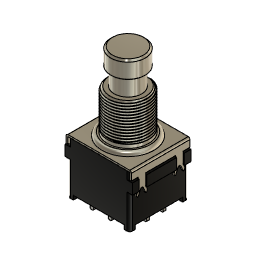
SF17010F-0302-21R-L (Autodesk Fusion 360 design; units mm, degrees)
Autodesk Fusion 360 part; units mm, degrees
ref_plane "WorkPlane1" through (0, 0, 1.2) normal (0, 0, 1) x (1, 0, 0)
sketch "Sketch1" plane through (0, 0, 1.2) normal (0, 0, 1) x (1, 0, 0)
  line L0 (-50, 50) -> (-30.4, 50)
  line L1 (-30.4, 50) -> (-30.4, 33)
  line L2 (-30.4, 33) -> (-50, 33)
  line L3 (-50, 33) -> (-50, 50)
  line L4 (-50, 50) -> (-30.4, 33) construction
  line L5 (-30.4, 50) -> (-50, 33) construction
  line L6 (9, -8.5) -> (-9, -8.5)
  line L7 (-9, -8.5) -> (-9, 8.5)
  line L8 (-9, 8.5) -> (9, 8.5)
  line L9 (9, 8.5) -> (9, -8.5)
  line L10 (9, -8.5) -> (-9, 8.5) construction
  line L11 (-9, -8.5) -> (9, 8.5) construction
  line L12 (-9, 8.5) -> (-7.4, 8.5)
  line L13 (-7.4, 8.5) -> (-7.4, 6.9)
  line L14 (-7.4, 6.9) -> (-9, 6.9)
  line L15 (-9, 6.9) -> (-9, 8.5)
  line L16 (-9, -8.5) -> (-7.4, -8.5)
  line L17 (-7.4, -8.5) -> (-7.4, -6.9)
  line L18 (-7.4, -6.9) -> (-9, -6.9)
  line L19 (-9, -6.9) -> (-9, -8.5)
  line L20 (9, -8.5) -> (7.4, -8.5)
  line L21 (7.4, -8.5) -> (7.4, -6.9)
  line L22 (7.4, -6.9) -> (9, -6.9)
  line L23 (9, -6.9) -> (9, -8.5)
  line L24 (9, 8.5) -> (7.4, 8.5)
  line L25 (7.4, 8.5) -> (7.4, 6.9)
  line L26 (7.4, 6.9) -> (9, 6.9)
  line L27 (9, 6.9) -> (9, 8.5)
  line L28 (1.7, -0.4) -> (-1.7, -0.4)
  line L29 (-1.7, -0.4) -> (-1.7, 0.4)
  line L30 (-1.7, 0.4) -> (1.7, 0.4)
  line L31 (1.7, 0.4) -> (1.7, -0.4)
  line L32 (1.7, -0.4) -> (-1.7, 0.4) construction
  line L33 (-1.7, -0.4) -> (1.7, 0.4) construction
  line L34 (-3.6, -4.4) -> (-3.6, -5.2)
  line L35 (-7, -4.4) -> (-3.6, -4.4)
  line L36 (-7, -5.2) -> (-7, -4.4)
  line L37 (-3.6, -5.2) -> (-7, -5.2)
  line L38 (1.7, -4.4) -> (1.7, -5.2)
  line L39 (-1.7, -4.4) -> (1.7, -4.4)
  line L40 (-1.7, -5.2) -> (-1.7, -4.4)
  line L41 (1.7, -5.2) -> (-1.7, -5.2)
  line L42 (7, -4.4) -> (7, -5.2)
  line L43 (3.6, -4.4) -> (7, -4.4)
  line L44 (3.6, -5.2) -> (3.6, -4.4)
  line L45 (7, -5.2) -> (3.6, -5.2)
  line L46 (-3.6, 0.4) -> (-3.6, -0.4)
  line L47 (-7, 0.4) -> (-3.6, 0.4)
  line L48 (-7, -0.4) -> (-7, 0.4)
  line L49 (-3.6, -0.4) -> (-7, -0.4)
  line L50 (7, 0.4) -> (7, -0.4)
  line L51 (3.6, 0.4) -> (7, 0.4)
  line L52 (3.6, -0.4) -> (3.6, 0.4)
  line L53 (7, -0.4) -> (3.6, -0.4)
  line L54 (-3.6, 5.2) -> (-3.6, 4.4)
  line L55 (-7, 5.2) -> (-3.6, 5.2)
  line L56 (-7, 4.4) -> (-7, 5.2)
  line L57 (-3.6, 4.4) -> (-7, 4.4)
  line L58 (1.7, 5.2) -> (1.7, 4.4)
  line L59 (-1.7, 5.2) -> (1.7, 5.2)
  line L60 (-1.7, 4.4) -> (-1.7, 5.2)
  line L61 (1.7, 4.4) -> (-1.7, 4.4)
  line L62 (7, 5.2) -> (7, 4.4)
  line L63 (3.6, 5.2) -> (7, 5.2)
  line L64 (3.6, 4.4) -> (3.6, 5.2)
  line L65 (7, 4.4) -> (3.6, 4.4)
  line L66 (0, 4.4) -> (0, 0.4) construction
  line L67 (0, -0.4) -> (0, -4.4) construction
  line L68 (7.5, 1.975) -> (-7.5, 1.975)
  line L69 (-7.5, 1.975) -> (-7.5, 2.825)
  line L70 (-7.5, 2.825) -> (7.5, 2.825)
  line L71 (7.5, 2.825) -> (7.5, 1.975)
  line L72 (7.5, 1.975) -> (-7.5, 2.825) construction
  line L73 (-7.5, 1.975) -> (7.5, 2.825) construction
  line L74 (7.5, -2.825) -> (-7.5, -2.825)
  line L75 (-7.5, -2.825) -> (-7.5, -1.975)
  line L76 (-7.5, -1.975) -> (7.5, -1.975)
  line L77 (7.5, -1.975) -> (7.5, -2.825)
  line L78 (7.5, -2.825) -> (-7.5, -1.975) construction
  line L79 (-7.5, -2.825) -> (7.5, -1.975) construction
  point P0 (-40.2, 41.5)
  point P1 (0, 2.4)
  point P2 (0, -2.4)
  point P3 (0, 2.4)
  point P4 (0, -2.4)
  dimension "d1" = 19.6
  dimension "d2" = 17
  dimension "d3" = 18
  dimension "d4" = 17
  dimension "d5" = 1.6
  dimension "d6" = 1.6
  dimension "d7" = 1.6
  dimension "d8" = 1.6
  dimension "d9" = 1.6
  dimension "d10" = 1.6
  dimension "d11" = 1.6
  dimension "d12" = 1.6
  dimension "d13" = 3.4
  dimension "d14" = 0.8
  dimension "d17" = 5.3
  dimension "d18" = 4.8
  dimension "d19" = 15
  dimension "d20" = 0.85
  dimension "d21" = 15
  dimension "d22" = 0.85
  constraint horizontal L0
  constraint vertical L1
  constraint horizontal L2
  constraint vertical L3
  constraint midpoint L4 P0
  constraint horizontal L6
  constraint perpendicular L6 L7
  constraint parallel L6 L8
  constraint parallel L7 L9
  constraint coincident L10 origin
  constraint coincident L11 origin
  constraint horizontal L12
  constraint vertical L13
  constraint horizontal L14
  constraint vertical L15
  constraint horizontal L16
  constraint vertical L17
  constraint horizontal L18
  constraint vertical L19
  constraint horizontal L20
  constraint vertical L21
  constraint horizontal L22
  constraint vertical L23
  constraint horizontal L24
  constraint vertical L25
  constraint horizontal L26
  constraint vertical L27
  constraint horizontal L28
  constraint perpendicular L28 L29
  constraint parallel L28 L30
  constraint parallel L29 L31
  constraint coincident L32 origin
  constraint coincident L33 origin
  constraint midpoint L61 L66.start
  constraint midpoint L30 L66.end
  constraint midpoint L66 P3
  constraint midpoint L28 L67.start
  constraint midpoint L39 L67.end
  constraint midpoint L67 P4
  constraint horizontal L68
  constraint perpendicular L68 L69
  constraint parallel L68 L70
  constraint parallel L69 L71
  constraint coincident L72 P3
  constraint coincident L73 P3
  constraint coincident P3 P1
  constraint horizontal L74
  constraint perpendicular L74 L75
  constraint parallel L74 L76
  constraint parallel L75 L77
  constraint coincident L78 P4
  constraint coincident L79 P4
  constraint coincident P4 P2
  measures "d1" distance of L0.start L0.end
  measures "d2" distance of L0.start L2.end
  measures "d3" distance of L7.end L8.end
  measures "d4" distance of L6.end L7.end
  measures "d5" distance of L7.end L12.end
  measures "d6" distance of L7.end L14.end
  measures "d7" distance of L6.end L16.end
  measures "d8" distance of L6.end L18.end
  measures "d9" distance of L6.start L20.end
  measures "d10" distance of L6.start L22.end
  measures "d11" distance of L8.end L24.end
  measures "d12" distance of L8.end L26.end
  measures "d13" distance of L29.end L30.end
  measures "d14" distance of L28.end L29.end
  measures "d19" distance of L69.end L70.end
  measures "d20" distance of L68.end L69.end
  measures "d21" distance of L75.end L76.end
  measures "d22" distance of L74.end L75.end
extrude "Extrude1" add sketch "Sketch1" against normal blind 1.2 contours L6 L9 L20 L21 L22 L23 | L6 L7 L16 L17 L18 L19 | L8 L9 L24 L25 L26 L27 | L7 L8 L12 L13 L14 L15 makes body 1 at (7.9333, 7.4333, 1.2) makes body 2 at (7.9333, -7.9667, 1.2) makes body 3 at (-7.9333, 7.4333, 1.2) makes body 4 at (-8.4667, -7.9667, 1.2)
extrude "Extrude2" add sketch "Sketch1" against normal blind 1 separate body contours L68 L69 L70 L71 | L74 L75 L76 L77 makes body 5 at (2.5, -2.825, 0.8667) makes body 6 at (2.5, 1.975, 0.8667)
extrude "Extrude3" add sketch "Sketch1" along normal blind 14 contours L6 L9 L20 L21 L22 L23 | L6 L7 L8 L9 L13 L14 L17 L18 L21 L22 L25 L26 | L6 L7 L16 L17 L18 L19 | L8 L9 L24 L25 L26 L27 | L7 L8 L12 L13 L14 L15 | L28 L29 L30 L31 | L34 L35 L36 L37 | L38 L39 L40 L41 | L42 L43 L44 L45 | L46 L47 L48 L49 | L50 L51 L52 L53 | L54 L55 L56 L57 | L58 L59 L60 L61 | L62 L63 L64 L65 | L68 L69 L70 L71 | L74 L75 L76 L77 bodies 1 2 3 4 5 6
ref_plane "WorkPlane2" through (-8.2, -7.7, 9.8) normal (0, 0, -1) x (-1, 0, 0)
sketch "Sketch2" plane through (-8.7, -7.7, 9.8) normal (0, 0, -1) x (1, 0, 0)
  line L0 (17.7, 0.8) -> (17.7, -16.2)
  line L1 (17.7, -16.2) -> (-0.3, -16.2)
  line L2 (-0.3, -16.2) -> (-0.3, 0.8)
  line L3 (-0.3, 0.8) -> (17.7, 0.8)
  line L4 (8.7, -16.2) -> (8.7, 0.8) construction
  line L5 (-1.1, -16.2) -> (-0.3, -16.2)
  line L6 (-1.1, -14.25) -> (-0.3, -14.25)
  line L7 (-0.3, -7.7) -> (17.7, -7.7) construction
  line L8 (-1.1, -12.05) -> (-0.3, -12.05)
  line L9 (-1.1, -16.2) -> (-1.1, -14.25)
  line L10 (-1.1, 0.8) -> (-0.3, 0.8)
  line L11 (-1.1, 0.8) -> (-1.1, -1.15)
  line L12 (-1.1, -1.15) -> (-0.3, -1.15)
  line L13 (-1.1, -3.35) -> (-0.3, -3.35)
  line L14 (-1.1, -12.05) -> (-1.1, -3.35)
  line L15 (-1.1, -1.15) -> (-1.1, 0.8)
  line L16 (18.5, -1.15) -> (17.7, -1.15)
  line L17 (18.5, -12.05) -> (18.5, -3.35)
  line L18 (17.7, -16.2) -> (17.7, 0.8)
  line L19 (18.5, 0.8) -> (18.5, -1.15)
  line L20 (18.5, -3.35) -> (17.7, -3.35)
  line L21 (18.5, -1.15) -> (18.5, 0.8)
  line L22 (18.5, -12.05) -> (17.7, -12.05)
  line L23 (18.5, -16.2) -> (18.5, -14.25)
  line L24 (18.5, 0.8) -> (17.7, 0.8)
  line L25 (18.5, -16.2) -> (17.7, -16.2)
  line L26 (18.5, -14.25) -> (17.7, -14.25)
  point P0 (-0.3, 0.8)
  point P1 (17.7, -7.7)
  point P2 (17.7, 0.8)
  dimension "d31" = 9.8
  dimension "d32" = 1.95
  dimension "d33" = 2.2
  constraint vertical L9
  constraint midpoint L1 L4.start
  constraint midpoint L3 L4.end
  constraint coincident L1 L5.start
  constraint coincident L3 L10.start
  constraint coincident L1.end L2.start
  constraint coincident L2 L6.end
  constraint perpendicular L2 L6
  constraint midpoint L2 L7.start
  constraint midpoint L0 P1
  constraint coincident L8.start L9
  constraint coincident L2 L8.end
  constraint perpendicular L2 L8
  constraint collinear L9 L14
  constraint symmetric L1.end L7 P0
  constraint symmetric L5.start L7 L10.start
  constraint symmetric L6.start L7 L11.end
  constraint symmetric L6.end L7 L12.end
  constraint symmetric L7 L8.start L13.start
  constraint symmetric L7 L8.end L13.end
  constraint collinear L14 L15
  constraint symmetric L1.end L4 L0.end
  constraint symmetric P0 L4 P2
  constraint symmetric L5.start L4 L23.start
  constraint symmetric L10.start L4 L19.start
  constraint symmetric L4 L1.end L0.end
  constraint symmetric L4 L6.start L23.end
  constraint symmetric L4 L6.end L26.end
  constraint symmetric L4 L7.start P1
  constraint symmetric L4 L8.start L17.start
  constraint symmetric L4 L8.end L22.end
  constraint symmetric L4 P0 P2
  constraint symmetric L4 L11.end L16.start
  constraint symmetric L4 L12.end L16.end
  constraint symmetric L4 L10.start L19.start
  constraint symmetric L4 L13.start L17.end
  constraint symmetric L4 L13.end L20.end
  measures "d31" distance of L4 L9
  measures "d32" distance of L5 L6
  measures "d33" distance of L6 L8
extrude "Extrude4" add sketch "Sketch2" against normal blind 3.1 contours L0 L16 L18 L19 L21 L24 | L2 L10 L11 L12 L15 | L0 L17 L18 L20 L22 | L2 L8 L13 L14 | L0 L18 L23 L25 L26 | L2 L5 L6 L9 bodies 1
sketch "Sketch3" plane through (0, 0, 15.2) normal (0, 0, 1) x (-1, 0, 0)
  line L0 (-9, -8.5) -> (9, -8.5)
  line L1 (9, 8.5) -> (-9, 8.5)
  line L2 (9.5, -8.5) -> (9.5, 8.5)
  line L3 (-9.5, 8.5) -> (-9.5, -8.5)
  line L4 (9.5, -8.5) -> (9, -8.5)
  line L5 (9.5, 8.5) -> (9, 8.5)
  line L6 (-9.5, 8.5) -> (-9, 8.5)
  line L7 (-9.5, -8.5) -> (-9, -8.5)
  line L8 (9, -8.5) -> (9, 8.5)
  line L9 (-9, 8.5) -> (-9, -8.5)
  constraint coincident L0.end L4.end
  constraint coincident L1.start L5.end
  constraint coincident L1.end L6.end
  constraint coincident L0.start L7.end
extrude "Extrude5" add sketch "Sketch3" along normal blind 0.5 separate body makes body 7
extrude "Extrude6" add sketch "Sketch3" against normal up to surface (1.95 mm away) contours L3 L6 L7 L9 | L2 L4 L5 L8 bodies 7
fillet "Fillet1" radius 0.5 2 edges at (-9.5, 0, 15.7) (9.5, 0, 15.7) on bodies 7
sketch "Sketch4" plane through (0, 0, 15.7) normal (0, 0, 1) x (-1, 0, 0)
  circle A0 centre (0, 0) radius 7.5
  line L0 (9, 8.5) -> (-9, 8.5)
  dimension "d44" = 1
  constraint coincident A0.centre origin
  measures "d44" distance of A0 L0
extrude "Extrude7" add sketch "Sketch4" along normal blind 1 bodies 7
fillet "Fillet2" radius 1 1 edges at (6.9925, 2.7121, 16.7) on bodies 7
sketch "Sketch5" plane through (0, 0, 16.7) normal (0, 0, 1) x (-1, 0, 0)
  circle A0 centre (0, 0) radius 6
  line L0 (-1, 0) -> (-1, -5.9161)
  line L1 (1, 0) -> (1, -5.9161)
  line L2 (1, -5) -> (-1, -5)
  line L3 (0, -5) -> (-0.75, -5)
  line L4 (-0.75, -5) -> (-0.75, -5.5)
  line L5 (-0.75, -5.5) -> (0.75, -5.5)
  line L6 (0.75, -5.5) -> (0.75, -5)
  line L7 (0.75, -5) -> (-0.1, -5)
  dimension "d49" = 12
  dimension "d50" = 2
  dimension "d51" = 1
  dimension "d52" = 0.75
  dimension "d53" = 0.5
  dimension "d54" = 1.5
  constraint coincident A0.centre origin
  constraint coincident A0 L0.end
  constraint vertical L0
  constraint coincident A0 L1.end
  constraint parallel L0 L1
  constraint coincident L1 L2.start
  constraint coincident L0 L2.end
  constraint perpendicular L0 L2
  constraint midpoint L2 L3.start
  constraint parallel L2 L3
  constraint perpendicular L2 L4
  constraint perpendicular L4 L5
  constraint coincident L2 L6.end
  constraint perpendicular L2 L6
  constraint coincident L3 L7.end
  constraint perpendicular L6 L7
  measures "d49" diameter of A0
  measures "d50" distance of L0 L1
  measures "d51" distance of A0 L2
  measures "d52" distance of L3.start L3.end
  measures "d53" distance of L3.end L4.end
  measures "d54" distance of L4.end L5.end
extrude "Extrude8" add sketch "Sketch5" along normal blind 0.8 contours L2 L3 L4 L5 L6 L7 bodies 7
fillet "Fillet3" radius 0.25 2 edges at (0.75, 5.25, 17.5) (-0.75, 5.25, 17.5) on bodies 7
extrude "Extrude9" add sketch "Sketch5" along normal blind 1 separate body contours A0 L0 L1 L2 L3 L7 makes body 8
sketch "Sketch8" plane through (0, 0, 17.7) normal (0, 0, 1) x (-1, 0, 0)
  circle A0 centre (0, 0) radius 6
  dimension "d72" = 12
  constraint coincident A0.centre origin
  measures "d72" diameter of A0
extrude "Extrude10" add sketch "Sketch8" 1 faces at (-0.1252, -2.3206, 17.7) along normal blind 10.5 separate body on bodies 8 makes body 9
thread "Thread1" "ISO Metric profile 12.0 M12x0.75 6g" major diameter 11.908 minor diameter 11.0445 pitch 0.75 angle 60 modelled right hand crest width 0.1036 on face at (-5.9925, 0.2991, 21.2) crest through (-5.954, 0, 17.5125) on bodies 9
sketch "Sketch7" plane through (0, 0, 28.2) normal (0, 0, 1) x (-1, 0, 0)
  circle A0 centre (0, 0) radius 6
  circle A1 centre (0, 0) radius 8
  dimension "d65" = 12
  dimension "d66" = 16
  constraint coincident A0.centre A1.centre
  measures "d65" diameter of A0
  measures "d66" diameter of A1
extrude "Extrude11" add sketch "Sketch7" against normal blind 0.8 separate body makes body 10
extrude "Extrude12" add sketch "Sketch7" along normal blind 1 contours A0 | A1 bodies 10
chamfer "Chamfer3" distance 0.8 angle 45 1 edges at (5.594, -2.1697, 28.2) on bodies 10
combine "Combine1" operation cut target body 9 tool bodies 10
move_body "Move1" bodies 9 to x (-0.5, 0.866025, 0) y (-0.866025, -0.5, 0) z (0, 0, 1) at (0, 0, 0)
extrude "Extrude13" cut sketch "Sketch5" along normal up to surface (11.5 mm away) contours A0 L0 L1 L2 L4 L5 L6 | L2 L3 L4 L5 L6 L7 bodies 9
combine "Combine2" operation add target body 9 tool bodies 8
sketch "Sketch9" plane through (0, 0, 28.2) normal (0, 0, 1) x (-1, 0, 0)
  circle A0 centre (0, 0) radius 4
  dimension "d75" = 8
  constraint coincident A0.centre origin
  measures "d75" diameter of A0
extrude "Extrude15" add 1 faces at (0, 1.3333, 16.7) along direction (0, 0, -1) up to surface (1.5 mm away) on bodies 9 bodies 9
extrude "Extrude16" cut sketch "Sketch9" against normal up to surface (13 mm away) bodies 7 9
combine "Combine3" operation cut target body 7 tool bodies 9 keep tools
sketch "Sketch10" plane through (0, 0, 15.2) normal (0, 0, -1) x (1, 0, 0)
  circle A0 centre (0, 0) radius 6
  dimension "d82" = 12
  constraint coincident A0.centre origin
  measures "d82" diameter of A0
extrude "Extrude17" cut sketch "Sketch10" against normal up to surface (1 mm away) bodies 7
extrude "Extrude18" add sketch "Sketch9" along normal blind 5 and the other way up to surface (13 mm away) separate body makes body 11
sketch "Sketch11" plane through (0, 0, 33.2) normal (0, 0, 1) x (-1, 0, 0)
  circle A0 centre (0, 0) radius 5
  dimension "d89" = 10
  constraint coincident A0.centre origin
  measures "d89" diameter of A0
extrude "Extrude19" add sketch "Sketch11" along normal blind 5 bodies 11
chamfer "Chamfer4" distance 0.5 angle 45 1 edges at (4.6616, 1.8081, 38.2) on bodies 11
chamfer "Chamfer4" distance 0.2 angle 45 1 edges at (4.6616, 1.8081, 33.2) on bodies 11
extrude "Extrude20" cut sketch "Sketch1" along normal blind 4 contours L28 L29 L30 L31 | L34 L35 L36 L37 | L38 L39 L40 L41 | L42 L43 L44 L45 | L46 L47 L48 L49 | L50 L51 L52 L53 | L54 L55 L56 L57 | L58 L59 L60 L61 | L62 L63 L64 L65 bodies 1
extrude "Extrude21" add sketch "Sketch1" along normal blind 4 separate body contours L28 L29 L30 L31 | L34 L35 L36 L37 | L38 L39 L40 L41 | L42 L43 L44 L45 | L46 L47 L48 L49 | L50 L51 L52 L53 | L54 L55 L56 L57 | L58 L59 L60 L61 | L62 L63 L64 L65 makes body 12 at (0.5667, -0.4, 2.5333) makes body 13 at (-4.7333, 4.4, 2.5333) makes body 14 at (0.5667, 4.4, 2.5333) makes body 15 at (0.5667, -5.2, 2.5333) makes body 16 at (4.7333, -0.4, 3.8667) makes body 17 at (-4.7333, -0.4, 2.5333) makes body 18 at (4.7333, 4.4, 3.8667) makes body 19 at (-4.7333, -5.2, 2.5333) makes body 20 at (4.7333, -5.2, 3.8667)
extrude "Extrude22" add 9 faces at (0.5667, 4.6667, 1.2) (5.8667, 4.6667, 1.2) (5.8667, -0.1333, 1.2) (0.5667, -0.1333, 1.2) (-4.7333, 4.6667, 1.2) (-4.7333, -0.1333, 1.2) (-4.7333, -4.9333, 1.2) (0.5667, -4.9333, 1.2) (5.8667, -4.9333, 1.2) along direction (0, 0, -1) blind 0.5 on bodies 12 13 14 15 16 17 18 19 20 bodies 14 12 13 15 16 17 18 19 20
sketch "Sketch12" plane through (0, 0, 0.7) normal (0, 0, -1) x (1, 0, 0)
  line L0 (0.5, -0.4) -> (-0.5, -0.4)
  line L1 (-0.5, -0.4) -> (-0.5, 0.4)
  line L2 (-0.5, 0.4) -> (0.5, 0.4)
  line L3 (0.5, 0.4) -> (0.5, -0.4)
  line L4 (0.5, -0.4) -> (-0.5, 0.4) construction
  line L5 (-0.5, -0.4) -> (0.5, 0.4) construction
  line L6 (-5.8, -5.2) -> (-4.8, -4.4) construction
  line L7 (-4.8, -5.2) -> (-5.8, -5.2)
  line L8 (-4.8, -4.4) -> (-4.8, -5.2)
  line L9 (-5.8, -4.4) -> (-4.8, -4.4)
  line L10 (-4.8, -5.2) -> (-5.8, -4.4) construction
  line L11 (-5.8, -5.2) -> (-5.8, -4.4)
  line L12 (-0.5, -5.2) -> (0.5, -4.4) construction
  line L13 (0.5, -5.2) -> (-0.5, -5.2)
  line L14 (0.5, -4.4) -> (0.5, -5.2)
  line L15 (-0.5, -4.4) -> (0.5, -4.4)
  line L16 (0.5, -5.2) -> (-0.5, -4.4) construction
  line L17 (-0.5, -5.2) -> (-0.5, -4.4)
  line L18 (4.8, -5.2) -> (5.8, -4.4) construction
  line L19 (5.8, -5.2) -> (4.8, -5.2)
  line L20 (5.8, -4.4) -> (5.8, -5.2)
  line L21 (4.8, -4.4) -> (5.8, -4.4)
  line L22 (5.8, -5.2) -> (4.8, -4.4) construction
  line L23 (4.8, -5.2) -> (4.8, -4.4)
  line L24 (-5.8, -0.4) -> (-4.8, 0.4) construction
  line L25 (-4.8, -0.4) -> (-5.8, -0.4)
  line L26 (-4.8, 0.4) -> (-4.8, -0.4)
  line L27 (-5.8, 0.4) -> (-4.8, 0.4)
  line L28 (-4.8, -0.4) -> (-5.8, 0.4) construction
  line L29 (-5.8, -0.4) -> (-5.8, 0.4)
  line L30 (4.8, -0.4) -> (5.8, 0.4) construction
  line L31 (5.8, -0.4) -> (4.8, -0.4)
  line L32 (5.8, 0.4) -> (5.8, -0.4)
  line L33 (4.8, 0.4) -> (5.8, 0.4)
  line L34 (5.8, -0.4) -> (4.8, 0.4) construction
  line L35 (4.8, -0.4) -> (4.8, 0.4)
  line L36 (-5.8, 4.4) -> (-4.8, 5.2) construction
  line L37 (-4.8, 4.4) -> (-5.8, 4.4)
  line L38 (-4.8, 5.2) -> (-4.8, 4.4)
  line L39 (-5.8, 5.2) -> (-4.8, 5.2)
  line L40 (-4.8, 4.4) -> (-5.8, 5.2) construction
  line L41 (-5.8, 4.4) -> (-5.8, 5.2)
  line L42 (-0.5, 4.4) -> (0.5, 5.2) construction
  line L43 (0.5, 4.4) -> (-0.5, 4.4)
  line L44 (0.5, 5.2) -> (0.5, 4.4)
  line L45 (-0.5, 5.2) -> (0.5, 5.2)
  line L46 (0.5, 4.4) -> (-0.5, 5.2) construction
  line L47 (-0.5, 4.4) -> (-0.5, 5.2)
  line L48 (4.8, 4.4) -> (5.8, 5.2) construction
  line L49 (5.8, 4.4) -> (4.8, 4.4)
  line L50 (5.8, 5.2) -> (5.8, 4.4)
  line L51 (4.8, 5.2) -> (5.8, 5.2)
  line L52 (5.8, 4.4) -> (4.8, 5.2) construction
  line L53 (4.8, 4.4) -> (4.8, 5.2)
  point P0 (-5.3, -4.8)
  point P1 (-5.3, -4.8)
  point P2 (0, -4.8)
  point P3 (0, -4.8)
  point P4 (5.3, -4.8)
  point P5 (5.3, -4.8)
  point P6 (-5.3, 0)
  point P7 (-5.3, 0)
  point P8 (5.3, 0)
  point P9 (5.3, 0)
  point P10 (-5.3, 4.8)
  point P11 (-5.3, 4.8)
  point P12 (0, 4.8)
  point P13 (0, 4.8)
  point P14 (5.3, 4.8)
  point P15 (5.3, 4.8)
  dimension "d100" = 1
  dimension "d101" = 0.8
  dimension "d104" = 5.3
  dimension "d105" = 4.8
  constraint horizontal L0
  constraint perpendicular L0 L1
  constraint parallel L0 L2
  constraint parallel L1 L3
  constraint coincident L4 origin
  constraint coincident L5 origin
  measures "d100" distance of L1.end L2.end
  measures "d101" distance of L0.end L1.end
extrude "Extrude23" add sketch "Sketch12" along normal up to surface (3.7 mm away) bodies 12 13 14 15 16 17 18 19 20
chamfer "Chamfer5" distance 0.4 angle 45 15 edges at (-5.8, 4.8, 0.7) (-4.8, 4.8, 0.7) (0.5, 0, 0.7) (-0.5, 0, 0.7) (-0.5, 4.8, 0.7) (0.5, 4.8, 0.7) (5.8, 0, 0.7) (0.5, -4.8, 0.7) (-0.5, -4.8, 0.7) (-5.8, 0, 0.7) (-4.8, 0, 0.7) (-5.8, -4.8, 0.7) (4.8, 4.8, 0.7) (5.8, 4.8, 0.7) (5.8, -4.8, 0.7) on bodies 12 13 14 15 16 17 18 19 20
fillet "Fillet6" radius 0.2 18 edges at (0.5, 0, -3) (-0.5, 0, -3) (-5.8, 4.8, -3) (-4.8, 4.8, -3) (0.5, 4.8, -3) (-0.5, 4.8, -3) (-0.5, -4.8, -3) (0.5, -4.8, -3) (4.8, 0, -3) (5.8, 0, -3) (-5.8, 0, -3) (-4.8, 0, -3) (4.8, 4.8, -3) (5.8, 4.8, -3) (-5.8, -4.8, -3) (-4.8, -4.8, -3) (4.8, -4.8, -3) (5.8, -4.8, -3) on bodies 12 13 14 15 16 17 18 19 20
sketch "Sketch14" plane through (-9, 0, 0) normal (-1, 0, 0) x (0, -1, 0)
  line L0 (-6.55, 9.8) -> (-6.55, 12.9)
  line L1 (-4.35, 9.8) -> (-4.35, 12.9)
  line L2 (8.5, 13.25) -> (-8.5, 13.25)
  line L3 (-6.55, 12.9) -> (-6.55, 13.25)
  line L4 (-4.35, 12.9) -> (-4.35, 13.25)
  line L5 (-6.55, 9.8) -> (-4.35, 9.8) construction
  line L6 (-5.4502, 10.2) -> (-5.4502, 7.9) construction
  line L7 (-6.6002, 8.194) -> (-5.8156, 9.9622)
  line L8 (-5.4502, 10.2) -> (-6.3831, 8.0977) construction
  line L9 (-6.3831, 8.0977) -> (-6.448, 8.1265) construction
  line L10 (-6.9561, 9.1178) -> (-6.55, 10.0331)
  line L11 (-6.6002, 8.194) -> (-6.6002, 8.194)
  arc A0 (-6.9561, 9.1178) -> (-6.6002, 8.194) centre (-6.3163, 8.8339) ccw
  line L12 (-3.9443, 9.1178) -> (-4.3504, 10.0331)
  arc A1 (-4.3002, 8.194) -> (-3.9443, 9.1178) centre (-4.5841, 8.8339) ccw
  line L13 (-4.3002, 8.194) -> (-5.0848, 9.9622)
  arc A2 (-5.0775, 9.9456) -> (-5.8156, 9.9622) centre (-5.45, 9.8) ccw
  line L14 (0, 13.25) -> (0, 7) construction
  line L15 (4.3002, 8.194) -> (5.0848, 9.9622)
  line L16 (6.6002, 8.194) -> (6.6002, 8.194)
  line L17 (3.9443, 9.1178) -> (4.3504, 10.0331)
  line L18 (4.35, 9.8) -> (4.35, 12.9)
  line L19 (6.55, 9.8) -> (6.55, 12.9)
  arc A3 (6.6002, 8.194) -> (6.9561, 9.1178) centre (6.3163, 8.8339) ccw
  line L20 (6.6002, 8.194) -> (5.8156, 9.9622)
  line L21 (5.4502, 10.2) -> (5.4502, 7.9) construction
  line L22 (6.55, 9.8) -> (4.35, 9.8) construction
  line L23 (5.4502, 10.2) -> (6.3831, 8.0977) construction
  line L24 (4.35, 12.9) -> (4.35, 13.25)
  line L25 (6.55, 12.9) -> (6.55, 13.25)
  line L26 (6.9561, 9.1178) -> (6.55, 10.0331)
  arc A4 (3.9443, 9.1178) -> (4.3002, 8.194) centre (4.5841, 8.8339) ccw
  line L27 (6.3831, 8.0977) -> (6.448, 8.1265) construction
  arc A5 (5.8156, 9.9622) -> (5.0775, 9.9456) centre (5.45, 9.8) ccw
  dimension "d123" = 0.8
  dimension "d127" = 2.3
  dimension "d128" = 1.15
  dimension "d130" = 0.7
  constraint coincident L0.end L3.start
  constraint coincident L2 L3.end
  constraint perpendicular L2 L3
  constraint coincident L1.end L4.start
  constraint coincident L2 L4.end
  constraint coincident L0.start L5.start
  constraint coincident L1.start L5.end
  constraint midpoint L5 A2.centre
  constraint perpendicular L5 L6
  constraint tangent L7 A2
  constraint coincident L6.start A2
  constraint parallel L7 L8
  constraint perpendicular L8 L9
  constraint collinear L7.start L8.end L9.end
  constraint parallel L7 L10
  constraint coincident L0 L10.end
  constraint tangent L10 A0
  constraint symmetric L6 L7.start A1.start
  constraint symmetric L6 L7.end L13.end
  constraint symmetric L6 L10.end L12.end
  constraint symmetric L6 L10.start L12.start
  constraint symmetric L6 A0 A1
  constraint coincident L13 A2.start
  constraint midpoint L2 L14.start
  constraint perpendicular L2 L14
  constraint symmetric L0.start L14 L19.start
  constraint symmetric L0.end L14 L19.end
  constraint symmetric L1.start L14 L18.start
  constraint symmetric L1.end L14 L18.end
  constraint symmetric L3.end L14 L25.end
  constraint symmetric L4.end L14 L24.end
  constraint symmetric L6.end L14 L21.end
  constraint symmetric L7.start L14 L16.start
  constraint symmetric L6.start L14 L21.start
  constraint symmetric L7.end L14 L20.end
  constraint symmetric L8.end L14 L23.end
  constraint symmetric L9.end L14 L27.end
  constraint symmetric L10.end L14 L26.end
  constraint symmetric L10.start L14 A3.end
  constraint symmetric A0 L14 A3
  constraint symmetric L12.start L14 L17.start
  constraint symmetric L12.end L14 L17.end
  constraint symmetric A1.start L14 L15.start
  constraint symmetric A1 L14 A4
  constraint symmetric L13.end L14 L15.end
  constraint symmetric A2 L14 A5
  constraint symmetric A2.start L14 A5.end
  measures "d123" diameter of A2
  measures "d127" distance of L6.start L8.end
  measures "d128" distance of L6 L7.start
  measures "d130" radius of A0
extrude "Extrude25" add sketch "Sketch14" along normal blind 0.5 separate body makes body 21 at (-9, 5.45, 12) makes body 22 at (-9, -5.45, 12)
mirror "Mirror1" about plane through (0, 0, 0) normal (1, 0, 0) of bodies 22 21 makes body 23 at (9, 5.45, 12) makes body 24 at (9, -5.45, 12)
combine "Combine4" operation cut target body 1 tool bodies 24 23 22 21 keep tools
combine "Combine5" operation add target body 7 tool bodies 21 23 24 22
fillet "Fillet7" radius 0.8 8 edges at (9, 8.5, 4.9) (9, -8.5, 4.9) (9, 8.5, 14.05) (9, -8.5, 14.05) (-9, 8.5, 14.05) (-9, 8.5, 4.9) (-9, -8.5, 14.05) (-9, -8.5, 4.9) on bodies 1
equation "d17 = ( 10.6 / 2 ) * 1 mm"
equation "d18 = ( 9.6 / 2 ) * 1 mm"
equation "d31 = ( 19.6 / 2 ) * 1 mm"
equation "d52 = ( 1.5 / 2 ) * 1 mm"
equation "d104 = ( 10.6 / 2 ) * 1 mm"
equation "d105 = ( 9.6 / 2 ) * 1 mm"
equation "d128 = ( 2.3 / 2 ) * 1 mm"
